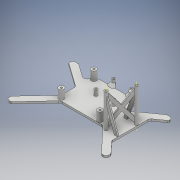
# Autodesk Inventor part: Holder_UP-Squared_IMU
Saved by Autodesk Inventor 2018 (Build 220112000, 112)
## iProperties
Created: 2018-07-31
Part Number: Holder_UP-Squared_IMU
Material: Generic
Document SubType Name: Modeling
Designer: Tsche
Density: 1 g/cm^3
Appearance: Default
Author: Tsche
Autodesk Inventor part; units mm, degrees
ref_plane "YZ Plane" through (0, 0, 0) normal (1, 0, 0) x (0, 1, 0)
ref_plane "XZ Plane" through (0, 0, 0) normal (0, 1, 0) x (-1, 0, 0)
sketch "Sketch1" plane through (0, 0, 0) normal (0, 0, 1) x (1, 0, 0)
  line L0 (-58.3, 45) -> (27.3, 45) construction
  line L1 (27.3, 45) -> (27.3, -45) construction
  line L2 (27.3, -45) -> (-58.3, -45) construction
  line L3 (-58.3, -45) -> (-58.3, 45) construction
  line L4 (37.3, 22) -> (58.3, 22) construction
  line L5 (58.3, 22) -> (58.3, -22) construction
  line L6 (58.3, -22) -> (37.3, -22) construction
  line L7 (37.3, -22) -> (37.3, 22) construction
  circle A0 centre (55.8, 14.9433) radius 1.4
  circle A1 centre (39.8, -14.9433) radius 1.4
  line L8 (37.3, 22) -> (58.3, -22) construction
  line L9 (37.3, -22) -> (58.3, 22) construction
  line L10 (39.8, -14.9433) -> (55.8, 14.9433) construction
  line L11 (-34.8, 41.5) -> (23.2, 41.5) construction
  line L12 (23.2, 41.5) -> (23.2, -7.5) construction
  line L13 (23.2, -7.5) -> (-34.8, -7.5) construction
  line L14 (-34.8, -7.5) -> (-34.8, 41.5) construction
  circle A2 centre (-34.8, 41.5) radius 2.5
  circle A3 centre (23.2, 41.5) radius 2.5
  circle A4 centre (-34.8, -7.5) radius 2.5
  circle A5 centre (23.2, -7.5) radius 2.5
  line L15 (-34.8, 41.5) -> (23.2, -7.5) construction
  line L16 (-34.8, -7.5) -> (23.2, 41.5) construction
  line L17 (-105, 0) -> (105, 0) construction
  line L18 (0, 71.872) -> (0, -70.312) construction
  line L19 (-75, 50) -> (75, 50) construction
  line L20 (75, 50) -> (75, -50) construction
  line L21 (75, -50) -> (-75, -50) construction
  line L22 (-75, -50) -> (-75, 50) construction
  line L23 (13.96, 49.06) -> (13.96, 22.39) construction
  line L24 (13.96, 22.39) -> (-12.71, 22.39) construction
  line L25 (-12.71, 22.39) -> (-12.71, 49.06) construction
  line L26 (-12.71, 49.06) -> (13.96, 49.06) construction
  arc A6 (13.96, 47.66) -> (15.36, 49.06) centre (13.96, 49.06) ccw
  circle A7 centre (13.96, 22.39) radius 1.4
  arc A8 (-12.71, 47.66) -> (-11.31, 49.06) centre (-12.71, 49.06) ccw
  circle A9 centre (-12.71, 22.39) radius 1.4
  line L27 (0, 26.2) -> (-12.71, 26.2) construction
  line L28 (-75, -50) -> (-68.1176, -50)
  line L29 (-68.1176, -50) -> (-31.7011, -11.5)
  line L30 (-31.7011, -11.5) -> (31.7011, -11.5)
  line L31 (31.7011, -11.5) -> (68.1176, -50)
  line L32 (75, -50) -> (75, -42.7238)
  line L33 (75, -42.7238) -> (58.3, -25.0684)
  line L34 (58.3, -25.0684) -> (58.3, 32.0314)
  line L35 (58.3, 32.0314) -> (75, 43.8709)
  line L36 (75, 43.8709) -> (75, 50)
  line L37 (75, 50) -> (66.3548, 50)
  line L38 (66.3548, 50) -> (27.2, 22.241)
  line L39 (27.2, 22.241) -> (27.2, 45.5)
  line L40 (27.2, 45.5) -> (20.02, 45.5)
  line L41 (-38.8, 45.5) -> (-38.8, 30.4649)
  line L42 (-38.8, 30.4649) -> (-66.3548, 50)
  line L43 (-75, 50) -> (-75, 43.8709)
  line L44 (-75, 50) -> (-66.3548, 50)
  line L45 (-75, 43.8709) -> (-38.8, 18.2068)
  line L46 (-38.8, 18.2068) -> (-38.8, -4.4527)
  line L47 (-38.8, -4.4527) -> (-75, -42.7238)
  line L48 (-75, -42.7238) -> (-75, -50)
  line L49 (-34.8, -7.5) -> (-75, -50) construction
  line L50 (68.1176, -50) -> (75, -50)
  line L51 (-75, 0) -> (75, 0) construction
  line L52 (-75, 50) -> (-34.8, 21.5) construction
  line L53 (-18.77, 45.5) -> (-15.21, 49.06)
  line L54 (-15.21, 49.06) -> (-10.21, 49.06)
  line L55 (-10.21, 49.06) -> (-6.65, 45.5)
  line L56 (-18.77, 45.5) -> (-38.8, 45.5)
  line L57 (-6.65, 45.5) -> (-18.77, 45.5) construction
  line L58 (7.9, 45.5) -> (11.46, 49.06)
  line L59 (11.46, 49.06) -> (12.56, 49.06)
  line L60 (16.46, 49.06) -> (20.02, 45.5)
  line L61 (7.9, 45.5) -> (-6.65, 45.5)
  line L62 (20.02, 45.5) -> (7.9, 45.5) construction
  circle A10 centre (-34.8, 41.5) radius 4
  circle A11 centre (23.2, 41.5) radius 4
  circle A12 centre (23.2, -7.5) radius 4
  circle A13 centre (-34.8, -7.5) radius 4
  arc A14 (-12.71, 46.56) -> (-10.21, 49.06) centre (-12.71, 49.06) ccw
  arc A15 (13.96, 46.56) -> (16.46, 49.06) centre (13.96, 49.06) ccw
  arc A16 (-14.11, 49.06) -> (-12.71, 47.66) centre (-12.71, 49.06) ccw
  arc A17 (-15.21, 49.06) -> (-12.71, 46.56) centre (-12.71, 49.06) ccw
  arc A18 (-11.31, 49.06) -> (-14.11, 49.06) centre (-12.71, 49.06) ccw
  arc A19 (-10.21, 49.06) -> (-15.21, 49.06) centre (-12.71, 49.06) ccw
  arc A20 (11.46, 49.06) -> (13.96, 46.56) centre (13.96, 49.06) ccw
  arc A21 (12.56, 49.06) -> (13.96, 47.66) centre (13.96, 49.06) ccw
  line L63 (15.36, 49.06) -> (16.46, 49.06)
  arc A22 (16.46, 49.06) -> (11.46, 49.06) centre (13.96, 49.06) ccw
  arc A23 (15.36, 49.06) -> (12.56, 49.06) centre (13.96, 49.06) ccw
  line L64 (12.56, 49.06) -> (15.36, 49.06)
  circle A24 centre (13.96, 22.39) radius 2.5
  circle A25 centre (-12.71, 22.39) radius 2.5
  circle A26 centre (23.2, 41.5) radius 1.4
  circle A27 centre (23.2, -7.5) radius 1.4
  circle A28 centre (-34.8, 41.5) radius 1.4
  circle A29 centre (-34.8, -7.5) radius 1.4
  circle A30 centre (55.8, 14.9433) radius 2.5
  circle A31 centre (39.8, -14.9433) radius 2.5
  point P0 (0, 0)
  point P1 (47.8, 0)
  point P2 (-58.3, 0)
  point P3 (47.8, 0)
  point P4 (13.96, 3.6346)
  point P5 (0, 22.39)
  dimension "d0" = 85.6
  dimension "d1" = 90
  dimension "d2" = 21
  dimension "d3" = 44
  dimension "d4" = 2.8
  dimension "d5" = 2.5
  dimension "d6" = 33.9
  dimension "d7" = 58
  dimension "d8" = 49
  dimension "d9" = 3.5
  dimension "d12" = 4.1
  dimension "d13" = 10
  dimension "d14" = 150
  dimension "d15" = 100
  dimension "d16" = 76.2
  dimension "d18" = 26.67
  dimension "d19" = 3.81
  dimension "d20" = 13.96
  dimension "d21" = 2.8
  dimension "d22" = 5
  dimension "d23" = 4
  dimension "d24" = 4
  dimension "d25" = 10
  dimension "d26" = 5
  dimension "d27" = 10
  dimension "d28" = 0
  dimension "d29" = 10
  dimension "d30" = 10
  dimension "d31" = 4
  dimension "d32" = 20
  dimension "d33" = 4
  dimension "d35" = 5
  dimension "d36" = 45
  dimension "d37" = 5
  dimension "d40" = 5
  dimension "d56" = 2.8
  dimension "d57" = 2.8
  dimension "d58" = 2.8
  dimension "d59" = 2.8
  dimension "d66" = 5
  dimension "d67" = 5
  constraints: 126 end point, 32 centre point, 26 point on line, 24 point on circle, 20 coincident, 20 parallel, 15 perpendicular, 9 equal radius, 7 horizontal, 6 collinear, 6 midpoint, 4 tangent, 2 concentric, 1 symmetric about line, 1 vertical, 7 other
  measures "d0" distance of L0.start L0.end
  measures "d1" distance of L2.end L0.start
  measures "d2" distance of L4.start L4.end
  measures "d3" distance of L4.end L5.end
  measures "d4" diameter of A0
  measures "d5" distance from line of L5 L10.end
  measures "d6" distance of L10.end L10.start
  measures "d7" distance of L11.start L11.end
  measures "d8" distance of L13.end L11.start
  measures "d9" distance between parallel lines of L0 L11
  measures "d12" distance between parallel lines of L1 L12
  measures "d13" distance between parallel lines of L1 L7
  measures "d14" distance of L19.start L19.end
  measures "d15" distance between parallel lines of L19 L21
  measures "d16" distance between parallel lines of L21 L27
  measures "d18" distance of L25.end L23.start
  measures "d19" distance between parallel lines of L27 L24
  measures "d20" distance between parallel lines of L18 L23
  measures "d21" diameter of A8
  measures "d22" distance between parallel lines of L19 L0
  measures "d23" distance between parallel lines of L30 L13
  measures "d24" distance between parallel lines of L46 L14
  measures "d25" distance between parallel lines of L47 L29
  measures "d26" distance between parallel lines of L29 L49
  measures "d27" distance between parallel lines of L33 L31
  measures "d28" distance between parallel lines of L5 L34
  measures "d29" distance between parallel lines of L42 L45
  measures "d30" distance between parallel lines of L38 L35
  measures "d31" distance between parallel lines of L39 L12
  measures "d32" distance from line of L11 L52.end
  measures "d33" distance between parallel lines of L40 L11
  measures "d35" distance of L53.end L54.end
  measures "d36" angle of L56 L53
  measures "d37" distance of L58.end L60.start
  measures "d40" diameter of A2
  measures "d56" diameter of A26
  measures "d57" diameter of A27
  measures "d58" diameter of A28
  measures "d59" diameter of A29
  measures "d66" diameter of A30
  measures "d67" diameter of A31
extrude "Extrusion1" add sketch "Sketch1" along normal blind 3 contours A0 | A1 | A21 L64 A6 | A6 L63 A15 A20 L59 A21 | A12 | A30 | L60 L40 A11 L39 L38 L37 L36 L35 L34 L33 L32 L50 L31 L30 L29 L28 L48 L47 L46 L45 L43 L44 L42 L41 A10 L56 L53 A17 A14 L55 L61 L58 A20 A15 | L40 L39 A11 | A11 | A14 A17 L54 A16 A8 | A8 A16 L54 | A10 L41 L56 | A10 | A7 | A9 | A13 | A24 | A25 | A31
extrude "Extrusion2" add sketch "Sketch1" along normal blind 15 contours A12 | A11 | A10 | A13
ref_plane "Work Plane2" through (0, 0, 11) normal (0, 0, 1) x (1, 0, 0)
ref_plane "Work Plane1" through (0, 0, 5) normal (0, 0, 1) x (1, 0, 0)
extrude "Extrusion3" add sketch "Sketch1" along normal up to surface (6 mm away) from surface at 5 contours A6 L63 A15 A20 L59 A21 | A23 L59 A22 L63 | A14 A17 L54 A16 A8 | L54 A18 A19
extrude "Extrusion4" add sketch "Sketch1" along normal up to surface (2 mm away) from surface at 3 contours A21 L64 A6 | A6 L63 A15 A20 L59 A21 | A14 A17 L54 A16 A8 | A8 A16 L54
chamfer "Chamfer1" distance 4 angle 45 2 edges at (-12.71, 46.56, 3) (13.96, 46.56, 3)
sketch "Sketch2" plane through (0, 0, 0) normal (1, 0, 0) x (0, 1, 0)
  line L0 (-10.312, 5) -> (61.872, 5) projected
  line L1 (51.56, 5) -> (51.56, 11) projected
  line L2 (49.06, 7) -> (49.06, 5) projected
  line L3 (49.06, 5) -> (51.56, 7.5)
  line L4 (51.56, 5) -> (49.06, 5)
  line L5 (51.56, 7.5) -> (51.56, 5)
  line L6 (45.5, 0) -> (45.5, 3) projected
  point P0 (0, 0)
  constraints: 6 end point, 1 horizontal, 1 parallel, 1 perpendicular, 1 point on line
extrude "Extrusion5" cut sketch "Sketch2" along normal through all both and the other way through all
extrude "Extrusion6" add sketch "Sketch1" along normal up to surface (11 mm away) contours A24 | A25
extrude "Extrusion7" add sketch "Sketch1" along normal blind 1.5 from surface at 15 contours A2 | A3 | A4 | A5 | A12 | A11 | A10 | A13
extrude "Extrusion9" add sketch "Sketch1" against normal blind 0.15 from surface at 15 contours A2 | A3 | A4 | A5 | A12 | A11 | A10 | A13 | A26 | A27 | A28 | A29
extrude "Extrusion10" add sketch "Sketch1" along normal blind 37 and the other way blind 15 from surface at 16.5 contours A0 | A1 | A30 | A31
ref_plane "Work Plane3" through (39.8, -14.9433, 53.5) normal (0, 1, 0) x (-1, 0, 0)
sketch "Sketch4" plane through (39.8, -14.9433, 53.5) normal (0, 1, 0) x (-1, 0, 0)
  line L0 (0, 0) -> (-18.5, -50.5)
  line L1 (-18.5, -50.5) -> (-18.5, 0) construction
  line L2 (-13.5, -50.5) -> (-13.5, 0) construction
  line L3 (-13.5, -50.5) -> (-18.5, -50.5)
  line L4 (-18.5, -50.5) -> (-13.5, -50.5) projected
  line L5 (-13.5, -50.5) -> (0, -13.6486)
  line L6 (0, -13.6486) -> (0, 0)
  point P0 (39.8, -53.5)
  constraints: 8 end point, 2 perpendicular, 2 point on line, 1 parallel
extrude "Extrusion12" add sketch "Sketch4" along normal mid plane 2
ref_plane "Work Plane4" through (55.8, 14.9433, 53.5) normal (0, 1, 0) x (-1, 0, 0)
sketch "Sketch5" plane through (55.8, 14.9433, 53.5) normal (0, 1, 0) x (-1, 0, 0)
  line L0 (0, 0) -> (18.5, -50.5)
  line L1 (18.5, -50.5) -> (18.5, 0) construction
  line L2 (13.5, -50.5) -> (13.5, 0) construction
  line L3 (13.5, -50.5) -> (18.5, -50.5)
  line L4 (13.5, -50.5) -> (0, -13.6486)
  line L5 (0, -13.6486) -> (0, 0)
  line L6 (-2.5, -50.5) -> (-2.5, 0) projected
  point P0 (55.8, -53.5)
  constraints: 8 end point, 2 parallel, 2 point on line, 1 perpendicular
extrude "Extrusion13" add sketch "Sketch5" along normal mid plane 2
ref_plane "Work Plane5" through (39.8, -14.9433, 0) normal (-0.8816112, 0.4719764, 0) x (0, 0, 1)
sketch "Sketch6" plane through (39.8, -14.9433, 0) normal (-0.8816112, 0.4719764, 0) x (0, 0, 1)
  line L0 (53.5, 2.5) -> (53.5, -2.5) projected
  line L1 (53.5, 0) -> (32.2582, 16.95)
  line L2 (32.2582, 16.95) -> (53.5, 33.9)
  line L3 (53.5, 36.4) -> (53.5, 31.4) projected
  line L4 (45.4836, 0) -> (28.25, 13.7516)
  line L5 (3, 2.7273) -> (3, -5.2727) construction
  line L6 (3, 0) -> (24.2418, 16.95)
  line L7 (24.2418, 16.95) -> (3, 33.9)
  line L8 (3, 38.2315) -> (3, 31.3642) projected
  line L9 (11.0164, 33.9) -> (28.25, 20.1484)
  line L10 (28.25, 20.1484) -> (45.4836, 33.9)
  line L11 (28.25, 13.7516) -> (11.0164, 0)
  line L12 (11.0164, 33.9) -> (3, 33.9)
  line L13 (11.0164, 0) -> (3, 0)
  line L14 (45.4836, 0) -> (53.5, 0)
  line L15 (45.4836, 33.9) -> (53.5, 33.9)
  point P0 (0, -5.6105)
  point P1 (3, -4.7991)
  dimension "d78" = 5
  dimension "d79" = 5
  constraints: 24 end point, 6 collinear, 4 horizontal, 4 parallel, 2 midpoint, 2 point on line
  measures "d78" distance between parallel lines of L9 L7
  measures "d79" distance between parallel lines of L11 L6
extrude "Extrusion14" add sketch "Sketch6" along normal mid plane 2
extrude "Extrusion15" cut sketch "Sketch1" against normal blind 10 from surface at 53.5 contours A0 | A1
fillet "Fillet1" radius 4 4 edges at (-75, -50, 1.5) (-75, 50, 1.5) (75, 50, 1.5) (75, -50, 1.5)
fillet "Fillet2" radius 5 10 edges at (-31.7011, -11.5, 1.5) (31.7011, -11.5, 1.5) (58.3, -25.0684, 1.5) (58.3, 32.0314, 1.5) (27.2, 22.241, 1.5) (27.2, 45.5, 1.5) (-38.8, 45.5, 1.5) (-38.8, -4.4527, 1.5) (-38.8, 18.2068, 1.5) (-38.8, 30.4649, 1.5)
fillet "Fillet3" radius 2 8 edges at (68.1176, -50, 1.5) (75, -42.7238, 1.5) (75, 43.8709, 1.5) (66.3548, 50, 1.5) (-68.1176, -50, 1.5) (-75, -42.7238, 1.5) (-75, 43.8709, 1.5) (-66.3548, 50, 1.5)
body "Solid1"
